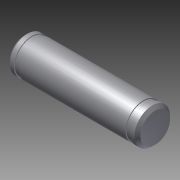
# Autodesk Inventor part: 13_0204_054
Saved by Autodesk Inventor 2012 SP1 (Build 160190100, 190)
## iProperties
Created: 2013-04-11
Part Number: 13_0204_054
Material: Default
Document SubType Name: Modeling
Designer: vogel
Density: 1 g/cm^3
Author: vogel
Autodesk Inventor part; units mm, degrees
ref_plane "YZ Plane" through (0, 0, 0) normal (1, 0, 0) x (0, 1, 0)
ref_plane "XZ Plane" through (0, 0, 0) normal (0, 1, 0) x (-1, 0, 0)
ref_plane "XY Plane" through (0, 0, 0) normal (0, 0, 1) x (1, 0, 0)
sketch "Skizze2" plane through (0, 0, 0) normal (0, 1, 0) x (-1, 0, 0)
  line L0 (15.4, 0) -> (-15.4, 0) projected
  line L1 (0, -0.6) -> (0, 3.6) projected
  line L2 (-11, 0) -> (11, 0)
  line L3 (11, 0) -> (11, 2.5)
  line L4 (-11, 2.5) -> (-11, 0)
  line L5 (-9, 3) -> (-9, 2.85)
  line L6 (-9, 2.85) -> (-9.8, 2.85)
  line L7 (-9.8, 2.85) -> (-9.8, 3)
  line L8 (9, 3) -> (9, 2.85)
  line L9 (9, 2.85) -> (9.8, 2.85)
  line L10 (9.8, 2.85) -> (9.8, 3)
  line L11 (-9.8, 3) -> (-10.5, 3)
  line L12 (10.5, 3) -> (9.8, 3)
  line L13 (9, 3) -> (-9, 3)
  line L14 (-11, 2.5) -> (-10.5, 3)
  line L15 (11, 2.5) -> (10.5, 3)
  point P0 (0, 0)
  point P1 (11, 3)
  point P2 (-11, 3)
  dimension "d3" = 6
  dimension "d4" = 5.7
  dimension "d5" = 22
  dimension "d6" = 18
  dimension "d7" = 0.8
  dimension "d8" = 0.5
  dimension "d9" = 0.5
  dimension "d10" = 0.5
  dimension "d11" = 0.5
  constraints: 28 end point, 6 parallel, 5 point on line, 3 collinear, 1 horizontal, 1 perpendicular, 3 other
  measures "d3" diameter of L12 L0
  measures "d4" diameter of L6 L0
  measures "d5" distance between parallel lines of L3 L4
  measures "d6" distance between parallel lines of L8 L5
  measures "d7" distance of L5.end L6.end
  measures "d8" distance of L4.start point (-11, 3)
  measures "d9" distance of L11.end point (-11, 3)
  measures "d10" distance of L3.end point (11, 3)
  measures "d11" distance of L12.start point (11, 3)
revolve "Umdrehung1" add sketch "Skizze2" angle 360 about axis through (-10, 0, 0) along (1, 0, 0)
equation "\"d9\" = d8"
equation "\"d10\" = d8"
equation "\"d11\" = d10"
